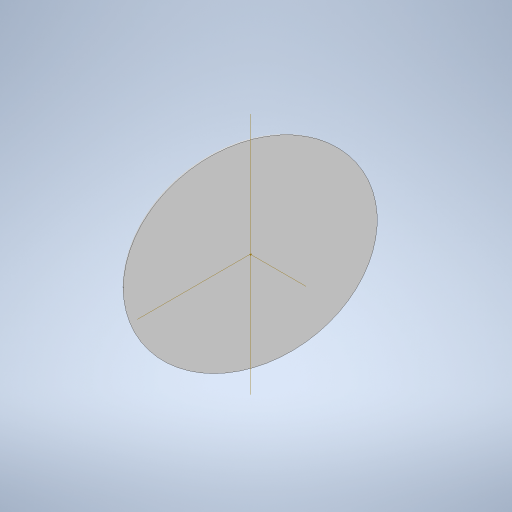
# Autodesk Inventor part: Disk
Saved by Autodesk Inventor 2023.2 (Build 272271030, 271C)
## iProperties
Created: 2023-02-26
Part Number: Disk
Material: Generisch
Document SubType Name: Modeling
Designer: mehan
Density: 1 g/cm^3
Appearance: Vorgabe
Author: mehan
Autodesk Inventor part; units mm, degrees
ref_plane "YZ Plane" through (0, 0, 0) normal (1, 0, 0) x (0, 1, 0)
ref_plane "XZ Plane" through (0, 0, 0) normal (0, 1, 0) x (-1, 0, 0)
ref_plane "XY Plane" through (0, 0, 0) normal (0, 0, 1) x (1, 0, 0)
sketch "Skizze3" plane through (0, 0, 0) normal (0, 1, 0) x (-1, 0, 0)
  line L0 (0, 0) -> (104.3161, 286.6062)
  line L1 (0, 0) -> (305, 0) construction
  line L2 (0, 0) -> (305, 0) construction
  line L3 (0, 0) -> (52.4348, -19.0847)
  line L4 (0, 0) -> (55.8, 0) construction
  ellipse E0 centre (0, 0) end of major axis (52.4348, -19.0847) minor radius 305 (52.4348, -19.0847) -> (104.3161, 286.6062) ccw
  dimension "d3" = 305
  dimension "d4" = 70
  dimension "d8" = 55.8
  dimension "d9" = 20
  constraints: 10 end point, 3 horizontal, 2 equal length, 1 coincident, 4 other
  measures "d3" distance of L0.start L0.end
  measures "d4" angle of L1 L0
  measures "d8" distance of L0.start L3.end
  measures "d9" angle of L3 L4
revolve "Umdrehung1" add sketch "Skizze3" angle 360 about axis through (0, 0, 0) along (-0.9396926, 0, -0.3420201)
